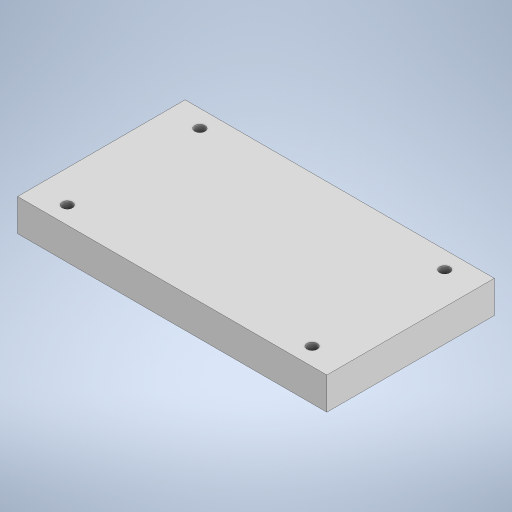
# Autodesk Inventor part: body_under
Saved by Autodesk Inventor 2024.1 (Build 281209000, 209)
## iProperties
Created: 2024-10-10
Part Number: body_under
Material: 一般
Document SubType Name: Modeling
Designer: hibik
Density: 1 g/cm^3
Appearance: 既定
Author: hibik
Autodesk Inventor part; units mm, degrees
ref_plane "YZ Plane" through (0, 0, 0) normal (1, 0, 0) x (0, 1, 0)
ref_plane "XZ Plane" through (0, 0, 0) normal (0, 1, 0) x (-1, 0, 0)
ref_plane "XY Plane" through (0, 0, 0) normal (0, 0, 1) x (1, 0, 0)
sketch "スケッチ1" plane through (0, 0, 0) normal (0, 1, 0) x (-1, 0, 0)
  line L0 (-24, -13) -> (24, -13)
  line L1 (24, -13) -> (24, 13)
  line L2 (24, 13) -> (-24, 13)
  line L3 (-24, 13) -> (-24, -13)
  line L4 (-24, -13) -> (24, 13) construction
  line L5 (24, -13) -> (-24, 13) construction
  line L6 (-19, -10.2917) -> (19, -10.2917) construction
  line L7 (19, -10.2917) -> (19, 10.2917)
  line L8 (19, 10.2917) -> (-19, 10.2917) construction
  line L9 (-19, 10.2917) -> (-19, -10.2917)
  line L10 (-19, -10.2917) -> (19, 10.2917) construction
  line L11 (19, -10.2917) -> (-19, 10.2917) construction
  circle A0 centre (19, 10.2917) radius 0.8
  circle A1 centre (19, -10.2917) radius 0.8
  circle A2 centre (-19, -10.2917) radius 0.8
  circle A3 centre (-19, 10.2917) radius 0.8
  line L12 (-4, -10) -> (4, -10) construction
  line L13 (4, -10) -> (4, 10)
  line L14 (4, 10) -> (-4, 10) construction
  line L15 (-4, 10) -> (-4, -10)
  line L16 (-4, -10) -> (4, 10) construction
  line L17 (4, -10) -> (-4, 10) construction
  circle A4 centre (4, 10) radius 0.8
  circle A5 centre (-4, 10) radius 0.8
  circle A6 centre (-4, -10) radius 0.8
  circle A7 centre (4, -10) radius 0.8
  point P0 (0, 0)
  dimension "d3" = 48
  dimension "d4" = 26
  dimension "d5" = 5
  dimension "d6" = 1.6
  dimension "d7" = 3
  dimension "d8" = 4
  constraints: 36 end point, 8 centre point, 7 equal radius, 6 midpoint, 6 parallel, 5 coincident, 4 point on line, 3 horizontal, 3 perpendicular
  measures "d3" distance of L2.end L1.end
  measures "d4" distance of L1.end L0.end
  measures "d5" distance between parallel lines of L1 L7
  measures "d6" diameter of A0
  measures "d7" distance between parallel lines of L2 L14
  measures "d8" distance from line of point (0, 0) L13
extrude "押し出し1" add sketch "スケッチ1" along normal blind 5 contours L3 L2 L1 L0 | A4 | A5 | A6 | A7
